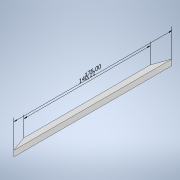
# Autodesk Inventor part: Top
Saved by Autodesk Inventor 2020.1 (Build 241239000, 239)
## iProperties
Created: 2019-12-12
Part Number: Top
Material: Generic
Document SubType Name: Modeling
Designer: super
Density: 1 g/cm^3
Appearance: Default
Author: super
Autodesk Inventor part; units mm, degrees
ref_plane "YZ Plane" through (0, 0, 0) normal (1, 0, 0) x (0, 1, 0)
ref_plane "XZ Plane" through (0, 0, 0) normal (0, 1, 0) x (-1, 0, 0)
ref_plane "XY Plane" through (0, 0, 0) normal (0, 0, 1) x (1, 0, 0)
sketch "Sketch1" plane through (0, 0, 0) normal (0, 1, 0) x (-1, 0, 0)
  line L0 (0, 0) -> (0, -175)
  line L1 (0, -175) -> (6.35, -175)
  line L2 (6.35, -175) -> (6.35, 0)
  line L3 (6.35, 0) -> (0, 0)
  dimension "d0" = 175
  dimension "d1" = 6.35
  constraints: 8 end point, 2 vertical, 1 horizontal, 1 perpendicular
  measures "d0" distance of L0.start L0.end
  measures "d1" distance of L0.end L1.end
extrude "Extrusion1" add sketch "Sketch1" along normal blind 6.35
sketch "Sketch2" plane through (0, 6.35, 0) normal (0, 1, 0) x (1, 0, 0)
  line L0 (-6.35, 0) -> (0, 0) projected
  line L1 (0, 0) -> (-6.35, 17.4465)
  line L2 (-6.35, 175) -> (-6.35, 0) projected
  line L3 (0, 0) -> (18.5662, 0) construction
  dimension "d4" = 110
  constraints: 4 end point, 1 equal length, 1 horizontal, 1 point on line
  measures "d4" angle of L3 L1
extrude "Extrusion2" cut sketch "Sketch2" against normal blind 6.35
sketch "Sketch3" plane through (0, 6.35, 0) normal (0, 1, 0) x (1, 0, 0)
  line L0 (0, 0) -> (0, 175) projected
  line L1 (0, 175) -> (-6.35, 157.5535)
  line L2 (-6.35, 175) -> (-6.35, 17.4465) projected
  line L3 (0, 175) -> (18.5662, 175) construction
  line L4 (0, 175) -> (-6.35, 175) projected
  line L5 (-6.35, 157.5535) -> (-6.35, 175)
  line L6 (-6.35, 175) -> (0, 175)
  dimension "d7" = 110
  constraints: 8 end point, 1 equal length, 1 horizontal, 1 perpendicular, 1 point on line, 1 vertical
  measures "d7" angle of L1 L3
extrude "Extrusion3" cut sketch "Sketch3" against normal blind 10
body "Solid1"
